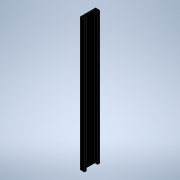
# Autodesk Inventor part: 14in-slide-pt_2
Saved by Autodesk Inventor 2020.1 (Build 241239000, 239)
## iProperties
Created: 2019-09-13
Part Number: 14in-slide-pt_2
Material: Aluminum 6061
Document SubType Name: Modeling
Designer: alpha
Density: 2.7 g/cm^3
Appearance: Anodized - Black
Author: alpha
Autodesk Inventor part; units mm, degrees
ref_plane "YZ Plane" through (0, 0, 0) normal (1, 0, 0) x (0, 1, 0)
ref_plane "XZ Plane" through (0, 0, 0) normal (0, 1, 0) x (-1, 0, 0)
ref_plane "XY Plane" through (0, 0, 0) normal (0, 0, 1) x (1, 0, 0)
sketch "Sketch1" plane through (0, 0, 0) normal (0, 1, 0) x (-1, 0, 0)
  line L0 (-4.7625, -17.4625) -> (4.7625, -17.4625)
  line L1 (4.7625, -17.4625) -> (4.7625, 17.4625)
  line L2 (4.7625, 17.4625) -> (-4.7625, 17.4625)
  line L3 (-4.7625, -17.4625) -> (4.7625, 17.4625) construction
  line L4 (4.7625, -17.4625) -> (-4.7625, 17.4625) construction
  line L5 (1.5875, -12.7) -> (1.5875, 12.7)
  line L6 (1.5875, 12.7) -> (-11.1125, -12.7) construction
  line L7 (-11.1125, 12.7) -> (1.5875, -12.7) construction
  line L8 (1.5875, 12.7) -> (-4.7625, 12.7)
  line L9 (1.5875, -12.7) -> (-4.7625, -12.7)
  line L10 (-4.7625, 12.7) -> (-4.7625, 17.4625)
  line L11 (-4.7625, -12.7) -> (-4.7625, -17.4625)
  point P0 (0, 0)
  point P1 (-4.7625, 0)
  dimension "d0" = 9.525
  dimension "d1" = 34.925
  dimension "d2" = 12.7
  dimension "d3" = 25.4
  constraints: 24 end point, 4 midpoint, 2 equal length, 1 horizontal, 1 perpendicular, 1 vertical
  measures "d0" distance of L2.end L1.end
  measures "d1" distance of L1.end L0.end
  measures "d2" distance of L5.start L6.end
  measures "d3" distance of L6.end L7.start
extrude "Extrusion1" add sketch "Sketch1" along normal blind 304.8
body "Solid1"
